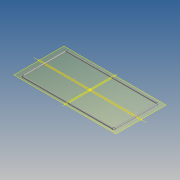
# Autodesk Inventor part: P048_BoitierCouvercleV4_joint
Saved by Autodesk Inventor 2021.3 (Build 253353000, 353)
## iProperties
Created: 2022-01-14
Part Number: P048_BoitierCouvercleV4_joint
Material: Générique
Document SubType Name: Modeling
Designer: gabri
Density: 1 g/cm^3
Appearance: Par défaut
Author: gabri
Autodesk Inventor part; units mm, degrees
sketch "Sketch2" plane through (0, 0, 0) normal (0, 0, 1) x (1, 0, 0)
  line L0 (94.5, -46.5) -> (-94.5, -46.5)
  line L1 (-96.5, -44.5) -> (-96.5, 44.5)
  line L2 (-94.5, 46.5) -> (94.5, 46.5)
  line L3 (96.5, 44.5) -> (96.5, -44.5)
  line L4 (96.5, -46.5) -> (-96.5, 46.5) construction
  line L5 (-96.5, -46.5) -> (96.5, 46.5) construction
  arc A0 (-94.5, 46.5) -> (-96.5, 44.5) centre (-94.5, 44.5) ccw
  arc A1 (96.5, 44.5) -> (94.5, 46.5) centre (94.5, 44.5) ccw
  arc A2 (94.5, -46.5) -> (96.5, -44.5) centre (94.5, -44.5) ccw
  arc A3 (-96.5, -44.5) -> (-94.5, -46.5) centre (-94.5, -44.5) ccw
  point P0 (0, 0)
  dimension "d0" = 193
  dimension "d1" = 93
  dimension "d2" = 2
  constraints: 12 end point, 8 point on circle, 8 point on line, 8 tangent, 4 centre point, 3 equal radius, 2 midpoint, 2 parallel, 1 horizontal, 1 perpendicular
  measures "d0" distance of L4.end L5.end
  measures "d1" distance of L5.start L4.end
  measures "d2" radius of A0
sketch "Sketch3" plane through (0, 0, 0) normal (0, 1, 0) x (-1, 0, 0)
  circle A0 centre (96.5, 0) radius 1.5
  point P0 (0, 0)
  dimension "d3" = 3
  constraints: 1 centre point, 1 coincident
  measures "d3" diameter of A0
sweep "Sweep1" add profiles "Sketch3" path "Sketch2" path curves L1 A3 L0 A2 L3 A1 L2 A0
body "Solid1"
